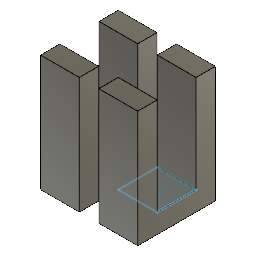
Fusion_BoxCAD (Autodesk Fusion 360 archive; units mm, degrees)
design "stopper"
Autodesk Fusion 360 part; units mm, degrees
sketch "スケッチ1" plane through (0, 0, 0) normal (0, 0, 1) x (1, 0, 0)
  line L0 (0, 0) -> (-30, 0)
  line L1 (-30, 0) -> (-30, 20)
  line L2 (-30, 20) -> (0, 20)
  line L3 (0, 20) -> (0, 0)
  line L4 (0, 5) -> (-25, 5)
  line L5 (-25, 5) -> (-25, 15)
  line L6 (-25, 15) -> (0, 15)
  line L7 (0, 15) -> (0, 5)
  dimension "d3" = 30
  dimension "d4" = 25
  dimension "d5" = 20
  constraint horizontal L0
  constraint vertical L1
  constraint horizontal L2
  constraint vertical L3
  constraint coincident L0.start L3.end
  constraint horizontal L4
  constraint vertical L5
  constraint horizontal L6
  constraint vertical L7
  constraint coincident L3 L4.start
  measures "d3" distance of L1.end L2.end
  measures "d4" distance of L5.end L6.end
  measures "d5" distance of L0.end L1.end
sketch "スケッチ2" plane through (0, 0, 0) normal (0, 0, 1) x (1, 0, 0)
  line L0 (0, 0) -> (-10, 0)
  line L1 (-10, 0) -> (-10, 20)
  line L2 (-10, 20) -> (0, 20)
  line L3 (0, 20) -> (0, 0)
  dimension "d6" = 10
  constraint horizontal L0
  constraint vertical L1
  constraint horizontal L2
  constraint vertical L3
  constraint coincident L0.start L3.end
  measures "d6" distance of L1.end L2.end
extrude "押し出し2" add sketch "スケッチ2" along normal blind 30 makes body 1
sketch "スケッチ3" plane through (0, 0, 0) normal (0, 1, 0) x (1, 0, 0)
sketch "スケッチ4" plane through (0, 0, 0) normal (0, 0, 1) x (1, 0, 0)
  line L0 (-10, 15, 5) -> (0, 15, 5)
  line L1 (0, 15, 5) -> (0, 5, 5)
  line L2 (0, 5, 5) -> (-10, 5, 5)
  line L3 (-10, 5, 5) -> (-10, 15, 5)
extrude "押し出し3" cut sketch "スケッチ4" along normal blind 25 contours L0 L1 L2 L3 in plane through (0, 0, 5) normal (0, 0, 1) bodies 1
copy_body "ボディのコピーと貼り付け2" bodies 1 makes body 2
move_body "移動2" bodies 2 to x (1, 0, 0) y (0, 1, 0) z (0, 0, 1) at (-15, 0, 0)

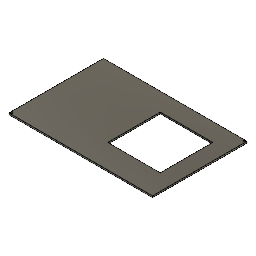
design "huta v3"
Autodesk Fusion 360 part; units mm, degrees
sketch "スケッチ1" plane through (0, 0, 0) normal (0, 0, 1) x (1, 0, 0)
  line L0 (0, 0) -> (-88, 0)
  line L1 (-88, 0) -> (-88, 58)
  line L2 (-88, 58) -> (0, 58)
  line L3 (0, 58) -> (0, 0)
  dimension "d10" = 58
  dimension "d11" = 88
  constraint horizontal L0
  constraint vertical L1
  constraint horizontal L2
  constraint vertical L3
  constraint coincident L0.start L3.end
  measures "d10" distance of L0.start L2.end
  measures "d11" distance of L1.end L2.end
extrude "押し出し1" add sketch "スケッチ1" along normal blind 1 makes body 1
sketch "スケッチ2" plane through (0, 0, 0) normal (0, 0, 1) x (1, 0, 0)
  line L0 (-10, 46.75) -> (-42, 46.75)
  line L1 (-42, 46.75) -> (-42, 14.75)
  line L2 (-42, 14.75) -> (-10, 14.75)
  line L3 (-10, 14.75) -> (-10, 46.75)
  constraint horizontal L0
  constraint vertical L1
  constraint horizontal L2
  constraint vertical L3
extrude "押し出し2" cut sketch "スケッチ2" along normal blind 1 bodies 1
move_face "面を移動1" by (-3, -3, 0) 1 faces at (-72.6667, 24.25, 1) on bodies 1
sketch "スケッチ3" plane through (0, 0, 0) normal (0, 0, 1) x (1, 0, 0)
  circle A0 centre (-87, 1) radius 0.5
extrude "押し出し3" cut sketch "スケッチ3" along normal blind 1 bodies 1
sketch "スケッチ4" plane through (0, 0, 0) normal (0, 0, 1) x (1, 0, 0)
  circle A0 centre (-1, 57) radius 0.5
extrude "押し出し4" cut sketch "スケッチ4" along normal blind 1 bodies 1
copy_body "ボディのコピーと貼り付け1" bodies 1 makes body 2
move_body "移動1" bodies 2 to x (1, 0, 0) y (0, 1, 0) z (0, 0, 1) at (0, 0, 0)

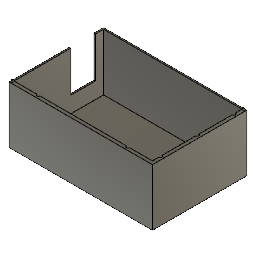
design "box v1"
Autodesk Fusion 360 part; units mm, degrees
sketch "スケッチ2" plane through (0, 0, 0) normal (0, 0, 1) x (1, 0, 0)
  line L0 (0, 0) -> (-85, 0)
  line L1 (-85, 0) -> (-85, 55)
  line L2 (-85, 55) -> (0, 55)
  line L3 (0, 55) -> (0, 0)
  constraint horizontal L0
  constraint vertical L1
  constraint horizontal L2
  constraint vertical L3
  constraint coincident L0.start L3.end
extrude "押し出し1" add sketch "スケッチ2" along normal blind 0.1
sketch "スケッチ3" plane through (0, 0, 0) normal (0, 0, 1) x (1, 0, 0)
  line L0 (0, 55) -> (2, 55)
  line L1 (2, 55) -> (2, -0.3729)
  line L2 (2, -0.3729) -> (0, -0.3729)
  line L3 (0, -0.3729) -> (0, 55)
  dimension "d3" = 2
  constraint horizontal L0
  constraint vertical L1
  constraint horizontal L2
  constraint vertical L3
  measures "d3" distance of L0.start L0.end
extrude "押し出し2" add sketch "スケッチ3" along normal blind 35
sketch "スケッチ4" plane through (0, 0, 0) normal (0, 0, 1) x (1, 0, 0)
  line L0 (-85, 55) -> (-86, 55)
  line L1 (-86, 55) -> (-86, 0)
  line L2 (-86, 0) -> (-85, 0)
  line L3 (-85, 0) -> (-85, 55)
  dimension "d6" = 1
  constraint horizontal L0
  constraint vertical L1
  constraint horizontal L2
  constraint vertical L3
  measures "d6" distance of L0.start L0.end
extrude "押し出し3" add sketch "スケッチ4" along normal blind 35
sketch "スケッチ5" plane through (0, 0, 0) normal (0, 0, 1) x (1, 0, 0)
  line L0 (-86, 55) -> (2, 55)
  line L1 (2, 55) -> (2, 56)
  line L2 (2, 56) -> (-86, 56)
  line L3 (-86, 56) -> (-86, 55)
  constraint horizontal L0
  constraint vertical L1
  constraint horizontal L2
  constraint vertical L3
sketch "スケッチ6" plane through (0, 0, 0) normal (0, 0, 1) x (1, 0, 0)
  line L0 (-86, 0) -> (2, 0)
  line L1 (2, 0) -> (2, -2)
  line L2 (2, -2) -> (-86, -2)
  line L3 (-86, -2) -> (-86, 0)
  constraint horizontal L0
  constraint vertical L1
  constraint horizontal L2
  constraint vertical L3
extrude "押し出し4" add sketch "スケッチ5" along normal blind 35
extrude "押し出し5" add sketch "スケッチ6" along normal blind 35
sketch "スケッチ7" plane through (0, 0, 0) normal (0, 0, 1) x (1, 0, 0)
  circle A0 centre (-15, 0) radius 1
extrude "押し出し6" cut sketch "スケッチ7" along normal blind 35
sketch "スケッチ8" plane through (0, 0, 0) normal (0, 0, 1) x (1, 0, 0)
  circle A0 centre (-70, 0) radius 1
extrude "押し出し7" cut sketch "スケッチ8" along normal blind 35
sketch "スケッチ9" plane through (0, 0, 0) normal (0, 0, 1) x (1, 0, 0)
  circle A0 centre (0, 5) radius 1
  circle A1 centre (0, 50) radius 1
  circle A2 centre (0, 27.5) radius 1
extrude "押し出し8" cut sketch "スケッチ9" along normal blind 35
sketch "スケッチ11" plane through (0, 0, 0) normal (0, 0, 1) x (1, 0, 0)
  circle A0 centre (-85, -1) radius 0.5
  circle A1 centre (1, 55) radius 0.5
extrude "押し出し9" add sketch "スケッチ11" along normal blind 36
sketch "スケッチ12" plane through (0, 0, 0) normal (0, 0, 1) x (1, 0, 0)
  line L0 (-86, 50, 10) -> (-85, 50, 10)
  line L1 (-85, 50, 10) -> (-85, 35, 10)
  line L2 (-85, 35, 10) -> (-86, 35, 10)
  line L3 (-86, 35, 10) -> (-86, 50, 10)
extrude "押し出し10" cut sketch "スケッチ12" along normal blind 30 contours L0 L1 L2 L3 in plane through (0, 0, 10) normal (0, 0, 1)
